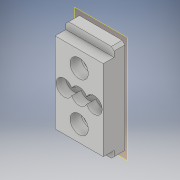
# Autodesk Inventor part: Omnivision_Objectivelens_mount
Saved by Autodesk Inventor 2019.4 (Build 234330000, 330)
## iProperties
Created: 2021-09-30
Part Number: Omnivision_Objectivelens_mount
Material: Generic
Document SubType Name: Modeling
Designer: diederichbenedict
Density: 1 g/cm^3
Appearance: Default
Author: diederichbenedict
Autodesk Inventor part; units mm, degrees
ref_plane "YZ Plane" through (0, 0, 0) normal (1, 0, 0) x (0, 1, 0)
ref_plane "XZ Plane" through (0, 0, 0) normal (0, 1, 0) x (-1, 0, 0)
ref_plane "XY Plane" through (0, 0, 0) normal (0, 0, 1) x (1, 0, 0)
ref_plane "Work Plane1" through (0, 0, 0) normal (0, 0, 1) x (1, 0, 0)
sketch "Sketch1" plane through (0, 0, 0) normal (0, 0, 1) x (1, 0, 0)
  circle A0 centre (0, -8.95) radius 4.2 projected
  circle A1 centre (0, 8.95) radius 4.2 projected
  circle A2 centre (0, 0) radius 1.4 projected
  circle A3 centre (3.9, 0) radius 0.1 projected
  line L0 (8.9, 16.9) -> (7.9, 17.9) projected
  line L1 (7.9, 17.9) -> (-7.9, 17.9) projected
  line L2 (-7.9, 17.9) -> (-8.9, 16.9) projected
  line L3 (-8.9, 16.9) -> (-8.9, -16.9) projected
  line L4 (-8.9, -16.9) -> (-7.9, -17.9) projected
  line L5 (-7.9, -17.9) -> (7.9, -17.9) projected
  line L6 (7.9, -17.9) -> (8.9, -16.9) projected
  line L7 (8.9, -16.9) -> (8.9, 16.9) projected
  point P0 (0, 0)
ref_plane "Work Plane2" through (-3.9, 5.05, 12.4) normal (0, 0, 1) x (1, 0, 0)
ref_plane "Work Plane3" through (-3.9, 5.05, 8) normal (0, 0, 1) x (1, 0, 0)
extrude "Extrusion1" add sketch "Sketch1" along normal up to surface (8 mm away) contours A0 | A1 | L7 L6 L5 L4 L3 L2 L1 L0
sketch "Sketch2" plane through (-7.9, 17.9, 8) normal (0, 0, 1) x (1, 0, 0)
  line L0 (16.8, -1) -> (16.8, -34.8) projected
  line L1 (15.8, 0) -> (16.8, -1) projected
  line L2 (0, 0) -> (15.8, 0) projected
  line L3 (-1, -1) -> (0, 0) projected
  line L4 (-1, -34.8) -> (-1, -1) projected
  line L5 (0, -35.8) -> (-1, -34.8) projected
  line L6 (15.8, -35.8) -> (0, -35.8) projected
  line L7 (16.8, -34.8) -> (15.8, -35.8) projected
  circle A0 centre (11.8, -17.9) radius 0.1 projected
  circle A1 centre (7.9, -17.9) radius 1.4 projected
  point P0 (7.9, -17.9)
  point P1 (13.4, -17.9)
  point P2 (2.4, -17.9)
  dimension "d2" = 5.5
  dimension "d3" = 5.5
  measures "d2" distance of point (13.4, -17.9) point (7.9, -17.9)
  measures "d3" distance of point (2.4, -17.9) point (7.9, -17.9)
hole "Hole1" at (5.5, 0, 8) at (-5.5, 0, 8) at (0, 0, 8) direction (0, 0, -1) diameter 2.9 end through all counterbore diameter 6 counterbore depth 3.5
sketch "Sketch3" plane through (0, 0, 0) normal (0, 0, -1) x (-1, 0, 0)
  circle A0 centre (0, 8.95) radius 3.9 construction
  circle A1 centre (0, -8.95) radius 3.9 construction
  circle A2 centre (0, 8.95) radius 3.375
  circle A3 centre (0, -8.95) radius 3.375
  point P0 (0, 0)
  dimension "d11" = 6.75
  dimension "d12" = 6.75
  constraints: 2 centre point, 2 coincident
  measures "d11" diameter of A2
  measures "d12" diameter of A3
extrude "Extrusion2" cut sketch "Sketch3" against normal blind 10
sketch "Sketch4" plane through (0, 0, 0) normal (0, 0, -1) x (-1, 0, 0)
  circle A0 centre (0, 8.95) radius 3.375 projected
  circle A1 centre (0, -8.95) radius 3.375 projected
  circle A2 centre (0, 8.95) radius 3.9
  circle A3 centre (0, -8.95) radius 3.9
  point P0 (0, 0)
  dimension "d15" = 7.8
  dimension "d16" = 7.8
  constraints: 2 centre point, 2 coincident
  measures "d15" diameter of A2
  measures "d16" diameter of A3
extrude "Extrusion3" cut sketch "Sketch4" against normal blind 4
sketch "Sketch5" plane through (0, 0, 0) normal (0, 0, -1) x (-1, 0, 0)
  circle A0 centre (0, 8.95) radius 3.9 projected
  circle A1 centre (0, 8.95) radius 3.9 projected
  circle A2 centre (0, -8.95) radius 3.9 projected
  circle A3 centre (-5.5, 0) radius 1.45 projected
  circle A4 centre (5.5, 0) radius 1.45 projected
  circle A5 centre (-3.9, 0) radius 0.1 projected
  line L0 (-8.9, 16.9) -> (-7.9, 17.9) projected
  line L1 (-8.9, -16.9) -> (-8.9, 16.9) projected
  line L2 (-7.9, -17.9) -> (-8.9, -16.9) projected
  line L3 (7.9, -17.9) -> (-7.9, -17.9) projected
  line L4 (8.9, -16.9) -> (7.9, -17.9) projected
  line L5 (8.9, 16.9) -> (8.9, -16.9) projected
  line L6 (7.9, 17.9) -> (8.9, 16.9) projected
  line L7 (-7.9, 17.9) -> (7.9, 17.9) projected
  line L8 (7.4, -16.2787) -> (7.2787, -16.4)
  line L9 (7.2787, -16.4) -> (-7.2787, -16.4)
  line L10 (-7.2787, -16.4) -> (-7.4, -16.2787)
  line L11 (-7.4, -16.2787) -> (-7.4, 16.2787)
  line L12 (-7.4, 16.2787) -> (-7.2787, 16.4)
  line L13 (-7.2787, 16.4) -> (7.2787, 16.4)
  line L14 (7.2787, 16.4) -> (7.4, 16.2787)
  line L15 (7.4, 16.2787) -> (7.4, -16.2787)
  point P0 (0, 0)
  dimension "d19" = 1.5
  constraints: 16 end point, 7 other
  measures "d19" distance between parallel lines of L5 L15
extrude "Extrusion4" cut sketch "Sketch5" against normal blind 3 contours A0 | A2 | A3 | A4 | L8 L9 L10 L11 L12 L13 L14 L15
sketch "Sketch6" plane through (-7.9, 17.9, 8) normal (0, 0, 1) x (1, 0, 0)
  circle A0 centre (7.9, -8.95) radius 3.375 projected
  circle A1 centre (7.9, -26.85) radius 3.375 projected
  arc A2 (5.15, -19.099) -> (10.65, -19.099) centre (7.9, -17.9) ccw projected
  arc A3 (5.15, -16.701) -> (5.15, -19.099) centre (2.4, -17.9) ccw projected
  arc A4 (10.65, -16.701) -> (5.15, -16.701) centre (7.9, -17.9) ccw projected
  arc A5 (10.65, -19.099) -> (10.65, -16.701) centre (13.4, -17.9) ccw projected
  line L0 (16.8, -1) -> (16.8, -34.8) projected
  line L1 (15.8, 0) -> (16.8, -1) projected
  line L2 (0, 0) -> (15.8, 0) projected
  line L3 (-1, -1) -> (0, 0) projected
  line L4 (-1, -34.8) -> (-1, -1) projected
  line L5 (0, -35.8) -> (-1, -34.8) projected
  line L6 (15.8, -35.8) -> (0, -35.8) projected
  line L7 (16.8, -34.8) -> (15.8, -35.8) projected
  line L8 (16.8, -34.8) -> (16.8, -1) projected
  line L9 (-1, 0) -> (16.8, 0)
  line L10 (16.8, 0) -> (16.8, -3)
  line L11 (16.8, -3) -> (-1, -3)
  line L12 (-1, -3) -> (-1, 0)
  line L13 (-1, -35.8) -> (16.8, -35.8)
  line L14 (16.8, -35.8) -> (16.8, -32.8)
  line L15 (16.8, -32.8) -> (-1, -32.8)
  line L16 (-1, -32.8) -> (-1, -35.8)
  dimension "d22" = 3
  dimension "d23" = 3
  constraints: 16 end point, 4 parallel, 3 point on line, 2 horizontal, 2 perpendicular
  measures "d22" distance of L9.end L10.end
  measures "d23" distance of L14.end L13.end
extrude "Extrusion5" cut sketch "Sketch6" against normal blind 4 contours L0 L11 L4 L3 L2 L1 | L1 L9 L10 | L0 L7 L6 L5 L4 L15 | L3 L12 L9 | L14 L13 L7 | L5 L13 L16
body "Solid1"
